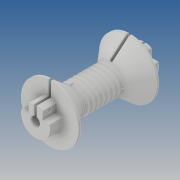
# Autodesk Inventor part: tambour
Saved by Autodesk Inventor 2019 (Build 230136000, 136)
## iProperties
Created: 2020-07-08
Part Number: tambour
Material: Générique
Document SubType Name: Modeling
Designer: Theo
Density: 1 g/cm^3
Appearance: Par défaut
Author: Theo
Autodesk Inventor part; units mm, degrees
ref_plane "YZ Plane" through (0, 0, 0) normal (1, 0, 0) x (0, 1, 0)
ref_plane "XZ Plane" through (0, 0, 0) normal (0, 1, 0) x (-1, 0, 0)
ref_plane "XY Plane" through (0, 0, 0) normal (0, 0, 1) x (1, 0, 0)
sketch "Esquisse1" plane through (0, 0, 0) normal (1, 0, 0) x (0, 1, 0)
  line L0 (0, 45.6) -> (0, -7.6) projected
  line L1 (10, 0) -> (10, 14.5)
  line L2 (10, 14.5) -> (20, 26.4175)
  line L3 (20, 26.4175) -> (20, 28)
  line L4 (3.125, 38) -> (3.125, 0)
  line L5 (3.125, 0) -> (10, 0)
  line L6 (-4, 0) -> (24, 0) projected
  line L7 (20, 28) -> (10, 28)
  line L8 (10, 28) -> (10, 38)
  line L9 (10, 38) -> (3.125, 38)
  point P0 (0, 0)
  dimension "d0" = 6.25
  dimension "d3" = 20
  dimension "d4" = 40
  dimension "d5" = 140
  dimension "d10" = 10
  dimension "d11" = 38
  dimension "d12" = 20
  dimension "d13" = 14.5
  constraints: 16 end point, 3 perpendicular, 1 collinear, 1 horizontal, 1 parallel, 1 vertical
  measures "d0" diameter of L4 L0
  measures "d3" diameter of L1 L0
  measures "d4" diameter of L3 L0
  measures "d5" angle of L2 L1
  measures "d10" distance of L7.end L8.end
  measures "d11" distance of L4.start L4.end
  measures "d12" diameter of L8 L0
  measures "d13" distance of L1.start L1.end
revolve "Révolution1" add sketch "Esquisse1" angle 360 about axis through (0, 0, 0) along (0, 0, -1)
sketch "Esquisse2" plane through (0, 0, 38) normal (0, 0, 1) x (1, 0, 0)
  circle A0 centre (0, 0) radius 3 projected
  circle A1 centre (0, 0) radius 25 projected
  line L0 (-0.8529, 33.1966) -> (0.8529, 33.1966)
  line L1 (0.8529, 33.1966) -> (0.8529, 1.3121)
  line L2 (0.8529, 1.3121) -> (-0.8529, 1.3121)
  line L3 (-0.8529, 1.3121) -> (-0.8529, 33.1966)
  line L4 (-0.8529, 33.1966) -> (0.8529, 1.3121) construction
  line L5 (0.8529, 33.1966) -> (-0.8529, 1.3121) construction
  point P0 (0, 17.2544)
  constraints: 12 end point, 2 midpoint, 2 parallel, 1 horizontal, 1 perpendicular
extrude "Extrusion1" cut sketch "Esquisse2" against normal blind 23.5 contours L1 L2 L3 A0 | A0 L3 A1 L1 | A1 L3 L0 L1 picked at (-0.0959, 1.8701) picked at (-0.0948, 10.3236)
sketch "Esquisse3" plane through (0, 0, 38) normal (0, 0, 1) x (1, 0, 0)
  arc A0 (-0.8529, 9.9636) -> (0.8529, 9.9636) centre (0, 0) ccw projected
  arc A1 (-0.8529, 3.0064) -> (0.8529, 3.0064) centre (0, 0) ccw projected
  line L0 (-4.8529, 13.318) -> (-12.0039, 13.318)
  line L1 (-12.0039, 13.318) -> (-12.0039, 2.8762)
  line L2 (-12.0039, 2.8762) -> (-4.8529, 2.8762)
  line L3 (-4.8529, 2.8762) -> (-4.8529, 13.318)
  line L4 (4.8529, 13.318) -> (14.6977, 13.318)
  line L5 (14.6977, 13.318) -> (14.6977, 2.8762)
  line L6 (14.6977, 2.8762) -> (4.8529, 2.8762)
  line L7 (4.8529, 2.8762) -> (4.8529, 13.318)
  line L8 (-0.8529, 3.0064) -> (-0.8529, 9.9636) projected
  line L9 (0.8529, 9.9636) -> (0.8529, 3.0064) projected
  constraints: 16 end point, 4 parallel, 2 horizontal, 2 perpendicular, 2 point on line
extrude "Extrusion2" cut sketch "Esquisse3" against normal up to surface (10 mm away) contours L3 L2 A0 | A0 L2 L1 L0 L3 | L6 L7 A0 | A0 L7 L4 L5 L6
sketch "Esquisse4" plane through (4.8529, 2.8762, 38) normal (1, 0, 0) x (0, 0, -1)
  line L0 (10, -22.8762) -> (10, 17.1056) projected
  line L1 (0, 0.1302) -> (0, 0.1302) projected
  line L2 (38, -6.0012) -> (38, 0.2488) projected
  line L3 (23.5, 0.1302) -> (0, 0.1302) projected
  line L4 (0, 0.1302) -> (23.5, 0.1302) projected
  line L5 (23.5, 0.1302) -> (23.5, 0.1302) projected
  point P0 (38, -2.8762)
  point P1 (5, 3.5)
  point P2 (0, 0.1238)
  point P3 (0, -5.8762)
  dimension "d18" = 5
  measures "d18" distance from line of point (5, 3.5) L0
hole "Perçage1" at (4.8529, 6.3762, 33) direction (-1, 0, 0) diameter 3.5 end through all
mirror "Symétrie1" about plane through (0, 0, 0) normal (0, 0, 1) of "Révolution1", "Extrusion1", "Extrusion2", "Perçage1"
sketch "Esquisse5" plane through (0, 0, 0) normal (1, 0, 0) x (0, 1, 0)
  line L0 (-10, 14.5) -> (-20, 26.4175) projected
  line L1 (-20, 26.4175) -> (-20, 28) projected
  line L2 (-20, 28) -> (-10, 28) projected
  line L3 (-10, 38) -> (-3.125, 38) projected
  line L4 (-3.125, 38) -> (-3.125, -38) projected
  line L5 (-3.125, -38) -> (-10, -38) projected
  line L6 (-10, -38) -> (-10, -28) projected
  line L7 (-10, -28) -> (-20, -28) projected
  line L8 (-20, -28) -> (-20, -26.4175) projected
  line L9 (-20, -26.4175) -> (-10, -14.5) projected
  line L10 (-10, -14.5) -> (-10, 14.5) projected
  circle A0 centre (11, 12.75) radius 1.75
  line L11 (-10, 14.5) -> (9.9636, 14.5) projected
  line L12 (0, 53.2) -> (0, -53.2) projected
  line L13 (-10, 28) -> (-10, 38) projected
  line L14 (10, -14.5) -> (3.125, -14.5) projected
  line L15 (3.125, -14.5) -> (3.125, 14.5) projected
  line L16 (3.125, 14.5) -> (10, 14.5) projected
  line L17 (10, 14.5) -> (10, -14.5) projected
  point P0 (0, 0)
  dimension "d26" = 3.5
  dimension "d27" = 1.75
  dimension "d28" = 11
  constraints: 1 centre point
  measures "d26" diameter of A0
  measures "d27" distance from line of A0.centre L11
  measures "d28" distance from line of A0.centre L12
coil "Hélicoïde1" sketch "Esquisse5" operation cut axis through (0, 0, 0) along (0, 0, -1) pitch 3.51 turns 7.264957 hand right contours A0 L17 | L17 A0
fillet "Congé1" radius 2 2 edges at (0, -10, -28) (0, -10, 28)
